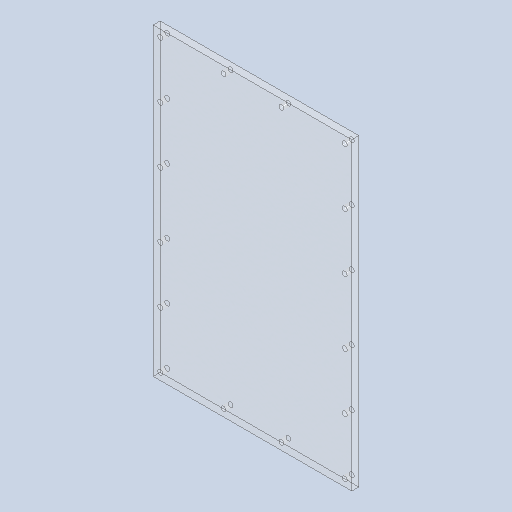
# Autodesk Inventor part: acrylic_for_PSI
Saved by Autodesk Inventor 2023 (Build 270158000, 158)
## iProperties
Created: 2023-05-18
Part Number: acrylic_for_PSI
Material: Aluminum 6061
Document SubType Name: Modeling
Designer: ASARe-DAQ-PC
Density: 2.7 g/cm^3
Appearance: Aluminum - Flat
Mass: 409.078 g
Surface Area: 650.538 cm^2
Volume: 151.51 cm^3
Author: ASARe-DAQ-PC
Autodesk Inventor part; units mm, degrees
ref_plane "YZ Plane" through (0, 0, 0) normal (1, 0, 0) x (0, 1, 0)
ref_plane "XZ Plane" through (0, 0, 0) normal (0, 1, 0) x (-1, 0, 0)
ref_plane "XY Plane" through (0, 0, 0) normal (0, 0, 1) x (1, 0, 0)
sketch "Sketch1" plane through (0, 0, 0) normal (0, 0, 1) x (1, 0, 0)
  line L0 (0, 0) -> (141, 0)
  line L1 (141, 0) -> (141, 216)
  line L2 (141, 216) -> (0, 216)
  line L3 (0, 216) -> (0, 0)
  dimension "d0" = 141
  dimension "d1" = 216
  constraints: 8 end point, 2 parallel, 1 horizontal, 1 perpendicular
  measures "d0" distance of L1.end L2.end
  measures "d1" distance of L0.end L1.end
extrude "Extrusion1" add sketch "Sketch1" along normal blind 5
sketch "Sketch2" plane through (0, 0, 5) normal (0, 0, 1) x (1, 0, 0)
  line L0 (141, 216) -> (0, 216) projected
  line L1 (0, 216) -> (0, 0) projected
  line L2 (141, 0) -> (141, 216) projected
  line L3 (0, 0) -> (141, 0) projected
  point P0 (5, 211)
  point P1 (136, 211)
  point P2 (136, 5)
  point P3 (5, 5)
  point P4 (5, 171)
  point P5 (136, 171)
  point P6 (5, 131)
  point P7 (136, 131)
  point P8 (50, 211)
  point P9 (50, 5)
  point P10 (91, 211)
  point P11 (91, 5)
  point P12 (5, 45)
  point P13 (136, 45)
  point P14 (5, 85)
  point P15 (136, 85)
  dimension "d11" = 5
  dimension "d12" = 5
  dimension "d13" = 5
  dimension "d14" = 5
  dimension "d15" = 5
  dimension "d16" = 5
  dimension "d17" = 5
  dimension "d18" = 5
  dimension "d35" = 40
  dimension "d42" = 45
  dimension "d49" = 45
  dimension "d56" = 40
  constraints: 2 horizontal, 2 vertical, 12 other
  measures "d11" distance from line of L0 point (5, 211)
  measures "d12" distance from line of L1 point (5, 211)
  measures "d13" distance from line of L2 point (136, 211)
  measures "d14" distance from line of point (136, 211) L0
  measures "d15" distance from line of L2 point (136, 5)
  measures "d16" distance from line of L3 point (136, 5)
  measures "d17" distance from line of L3 point (5, 5)
  measures "d18" distance from line of L1 point (5, 5)
  measures "d35" distance of point (5, 211) point (5, 171)
  measures "d42" distance of point (5, 211) point (50, 211)
  measures "d49" distance of point (136, 211) point (91, 211)
  measures "d56" distance of point (5, 5) point (5, 45)
hole "Hole1" at (5, 211, 5) at (136, 211, 5) at (136, 5, 5) at (5, 5, 5) at (5, 171, 5) at (136, 171, 5) at (5, 131, 5) at (136, 131, 5) at (50, 211, 5) at (50, 5, 5) at (91, 211, 5) at (91, 5, 5) at (5, 45, 5) at (136, 45, 5) at (5, 85, 5) at (136, 85, 5) direction (0, 0, -1) diameter 3.5 end through all
body "Solid1"
